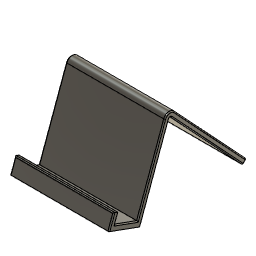
Phone+Holder (Autodesk Fusion 360 design; units mm, degrees)
Autodesk Fusion 360 part; units mm, degrees
sketch "Sketch1" plane through (0, 0, 0) normal (1, 0, 0) x (0, 1, 0) in component "stand"
  line L0 (-20.953, -72.187) -> (-7.2365, -34.5012)
  line L1 (-2.2234, -33.4813) -> (33.8703, -72.187)
  line L2 (-20.953, -72.187) -> (-32.2294, -68.0828)
  line L3 (-32.2294, -68.0828) -> (-30.5193, -63.3843)
  arc A0 (-2.2234, -33.4813) -> (-7.2365, -34.5012) centre (-4.4174, -35.5273) ccw
  line L4 (-4.0518, -35.1863) -> (32.042, -73.892)
  arc A1 (-4.0518, -35.1863) -> (-4.8873, -35.3562) centre (-4.4174, -35.5273) ccw
  line L5 (-19.4589, -75.3913) -> (-4.8873, -35.3562)
  line L6 (-19.4589, -75.3913) -> (-35.4336, -69.577)
  line L7 (-35.4336, -69.577) -> (-32.8685, -62.5293)
  line L8 (-32.8685, -62.5293) -> (-30.5193, -63.3843)
  line L9 (33.8703, -72.187) -> (32.042, -73.892)
  line L10 (-19.4589, -75.3913) -> (32.042, -73.892) construction
  point P0 (-20.953, -72.187)
  point P1 (-30.35, -68.7668)
  point P2 (-5.5621, -29.9009)
  dimension "d5" = 45
  dimension "d8" = 12
  dimension "d9" = 5
  dimension "d10" = 3
  dimension "d11" = 2.5
  dimension "d17" = 68.332
  constraint coincident P0 L0.start
  constraint perpendicular L0 L2
  constraint perpendicular L2 L3
  constraint coincident P2 L1
  constraint coincident P2 L0
  constraint tangent L1 A0
  constraint tangent L0 A0
  constraint perpendicular L3 L8
  measures "d5" distance of P0 P2
  measures "d8" distance of P0 L2.end
  measures "d9" distance of L2.end L3.end
  measures "d10" radius of A0
  measures "d17" angle of L0 L10
extrude "Extrude1" add sketch "Sketch1" along normal mid plane 50 in component "stand"
fillet "Fillet1" radius 0.5 20 edges at (25, 15.8235, -52.8342) (25, -5.0155, -32.5875) (25, -14.0948, -53.3441) (25, -12.1731, -55.3738) (25, -4.5171, -35.0373) (25, 13.9951, -54.5392) (25, -26.5912, -70.1349) (25, -34.1511, -66.0531) (25, -31.3743, -65.7336) (0, -30.5193, -63.3843) (0, -32.8685, -62.5293) (-25, 13.9951, -54.5392) (-25, -4.5171, -35.0373) (-25, -12.1731, -55.3738) (-25, -14.0948, -53.3441) (-25, -5.0155, -32.5875) (-25, 15.8235, -52.8342) (-25, -26.5912, -70.1349) (-25, -31.3743, -65.7336) (-25, -34.1511, -66.0531) in component "stand"
component "stand" placed x (1, 0, 0) y (0, 1, 0) z (0, 0, 1) at (0, 0, 0)
